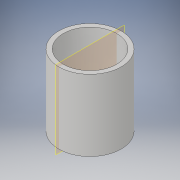
# Autodesk Inventor part: ExternalThreadedPart
Saved by Autodesk Inventor 2019.2 (Build 232265000, 265)
## iProperties
Created: 2018-12-30
Part Number: ExternalThreadedPart
Material: Generic
Document SubType Name: Modeling
Designer: steele
Density: 1 g/cm^3
Appearance: Default
Author: steele
Autodesk Inventor part; units mm, degrees
ref_plane "XZ Plane" through (0, 0, 0) normal (0, 1, 0) x (-1, 0, 0)
ref_plane "XY Plane" through (0, 0, 0) normal (0, 0, 1) x (1, 0, 0)
sketch "Sketch1" plane through (0, 0, 0) normal (0, 1, 0) x (-1, 0, 0)
  circle A0 centre (0, 0) radius 19.05
  circle A1 centre (0, 0) radius 22.225
  dimension "d0" = 38.1
  dimension "d1" = 44.45
  constraints: 2 centre point, 2 coincident
  measures "d0" diameter of A0
  measures "d1" diameter of A1
extrude "Extrusion1" add sketch "Sketch1" against normal blind 50.8
sketch "Sketch5" plane through (0, 0, 0) normal (1, 0, 0) x (0, 1, 0)
  line L0 (0, 19.05) -> (-50.8, 19.05) projected
  arc A0 (-25.4, 17.4625) -> (-25.4, 20.6375) centre (-25.4, 19.05) ccw
  line L1 (-25.4, 17.4625) -> (-25.4, 20.6375)
  line L2 (-25.4, 17.4625) -> (-25.4, 20.6375) construction
  point P0 (0, 0)
  constraints: 4 end point, 3 point on circle, 1 centre point, 1 midpoint, 1 perpendicular
revolve "Revolution2" add sketch "Sketch5" angle 360 about axis through (0, -25.4, 17.4625) along (0, 0, 1)
body "Solid1"
